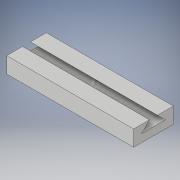
# Autodesk Inventor part: Test2
Saved by Autodesk Inventor 2018.2 (Build 222227000, 227)
## iProperties
Created: 2018-03-29
Part Number: Test2
Material: Generic
Document SubType Name: Modeling
Designer: martin
Density: 1 g/cm^3
Appearance: Default
Author: martin
Autodesk Inventor part; units mm, degrees
ref_plane "YZ Plane" through (0, 0, 0) normal (1, 0, 0) x (0, 1, 0)
ref_plane "XZ Plane" through (0, 0, 0) normal (0, 1, 0) x (-1, 0, 0)
ref_plane "XY Plane" through (0, 0, 0) normal (0, 0, 1) x (1, 0, 0)
sketch "Sketch1" plane through (0, 0, 0) normal (1, 0, 0) x (0, 1, 0)
  line L0 (0, 0) -> (0, -7.9375)
  line L1 (0, -7.9375) -> (6.35, -7.9375)
  line L2 (6.35, -7.9375) -> (6.35, -1.5875)
  line L3 (6.35, -1.5875) -> (3.175, -4.7625)
  line L4 (3.175, -4.7625) -> (3.175, 4.7625)
  line L5 (3.175, 4.7625) -> (6.35, 1.5875)
  line L6 (6.35, 1.5875) -> (6.35, 7.9375)
  line L7 (6.35, 7.9375) -> (0, 7.9375)
  line L8 (0, 7.9375) -> (0, 0)
  dimension "d0" = 7.9375
  dimension "d1" = 7.9375
  dimension "d2" = 6.35
  dimension "d3" = 6.35
  dimension "d4" = 6.35
  dimension "d5" = 6.35
  dimension "d6" = 9.525
  dimension "d7" = 45
  dimension "d8" = 45
  constraints: 18 end point, 5 perpendicular, 2 point on line, 1 parallel, 1 vertical
  measures "d0" distance of L0.start L0.end
  measures "d1" distance of L7.end L0.start
  measures "d2" distance of L0.end L1.end
  measures "d3" distance of L6.end L7.end
  measures "d4" distance of L1.end L2.end
  measures "d5" distance of L5.end L6.end
  measures "d6" distance of L3.end L4.end
  measures "d7" angle of L2 L3
  measures "d8" angle of L6 L5
extrude "Extrusion1" add sketch "Sketch1" along normal blind 50.8
sketch "Sketch2" plane through (0, 0, -7.9375) normal (0, 0, -1) x (-1, 0, 0)
  point P0 (0, 0)
body "Solid1"
